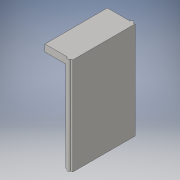
# Autodesk Inventor part: arduinocase
Saved by Autodesk Inventor 2016 (Build 200138000, 138)
## iProperties
Created: 2016-08-10
Part Number: arduinocase
Material: Generic
Document SubType Name: Modeling
Designer: Jorian Brusind
Density: 1 g/cm^3
Appearance: Default
Author: Jorian Brusind
Autodesk Inventor part; units mm, degrees
ref_plane "YZ Plane" through (0, 0, 0) normal (1, 0, 0) x (0, 1, 0)
ref_plane "XZ Plane" through (0, 0, 0) normal (0, 1, 0) x (-1, 0, 0)
ref_plane "XY Plane" through (0, 0, 0) normal (0, 0, 1) x (1, 0, 0)
sketch "Sketch1" plane through (0, 0, 0) normal (0, 1, 0) x (-1, 0, 0)
  line L0 (0, 0) -> (25.4, 0)
  line L1 (25.4, 0) -> (25.4, -57.15)
  line L2 (25.4, -57.15) -> (0, -57.15)
  line L3 (0, -57.15) -> (0, 0)
  dimension "d0" = 25.4
  dimension "d1" = 57.15
  constraints: 8 end point, 2 parallel, 1 horizontal, 1 perpendicular
  measures "d0" distance of L1.end L2.end
  measures "d1" distance of L0.end L1.end
extrude "Extrusion1" add sketch "Sketch1" along normal blind 88.9
sketch "Sketch2" plane through (0, 0, 0) normal (0, -1, 0) x (1, 0, 0)
  line L0 (0, 0) -> (-6.35, 0)
  line L1 (-25.4, 0) -> (0, 0) projected
  line L2 (-6.35, 0) -> (-6.35, -57.15)
  line L3 (0, -57.15) -> (-25.4, -57.15) projected
  line L4 (-6.35, 0) -> (-25.4, 0)
  line L5 (-25.4, -57.15) -> (-25.4, 0) projected
  line L6 (-25.4, -57.15) -> (-25.4, 0)
  line L7 (-25.4, -57.15) -> (-6.35, -57.15)
  dimension "d4" = 6.35
  constraints: 10 end point, 3 collinear, 2 point on line, 1 perpendicular
  measures "d4" distance of L0.start L0.end
extrude "Extrusion2" cut sketch "Sketch2" against normal blind 82.55
sketch "Sketch3" plane through (0, 88.9, 0) normal (0, 1, 0) x (1, 0, 0)
  line L0 (0, 0) -> (0, 57.15) projected
  line L1 (0, 57.15) -> (-3.175, 57.15)
  line L2 (-6.35, 57.15) -> (0, 57.15) projected
  arc A0 (-1.5875, 57.15) -> (-4.7625, 57.15) centre (-3.175, 57.15) ccw
  line L3 (-4.7625, 57.15) -> (0, 57.15)
  arc A1 (-4.7625, 0) -> (-1.5875, 0) centre (-3.175, 0) ccw
  line L4 (-4.7625, 0) -> (-1.5875, 0)
  line L5 (0, 0) -> (-3.175, 0)
  dimension "d12" = 3.175
  dimension "d13" = 3.175
  dimension "d17" = 3.175
  dimension "d18" = 3.175
  constraints: 8 end point, 4 point on circle, 2 centre point, 2 horizontal, 2 point on line, 1 coincident, 1 midpoint
  measures "d12" distance of L0.end L1.end
  measures "d13" diameter of A0
  measures "d17" diameter of A1
  measures "d18" distance of L0.start L5.end
extrude "Extrusion3" add sketch "Sketch3" against normal blind 88.9
body "Solid1"
